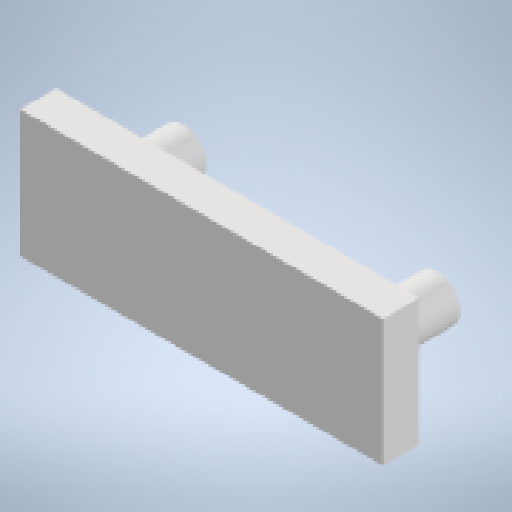
# Autodesk Inventor part: test_izbrisi
Saved by Autodesk Inventor 2023 (Build 270158000, 158)
## iProperties
Created: 2022-09-28
Part Number: test_izbrisi
Material: Generic
Document SubType Name: Modeling
Designer: simon
Density: 1 g/cm^3
Appearance: Default
Author: simon
Autodesk Inventor part; units mm, degrees
ref_plane "YZ Plane" through (0, 0, 0) normal (1, 0, 0) x (0, 1, 0)
ref_plane "XZ Plane" through (0, 0, 0) normal (0, 1, 0) x (-1, 0, 0)
ref_plane "XY Plane" through (0, 0, 0) normal (0, 0, 1) x (1, 0, 0)
sketch "Sketch2" plane through (0, 0, 0) normal (0, 0, 1) x (1, 0, 0)
  circle A0 centre (14, 0) radius 1.25 projected
  circle A1 centre (0, 0) radius 1.25 projected
  line L0 (-3, -3.5) -> (17, -3.5) projected
  line L1 (17, -3.5) -> (17, 3.5) projected
  line L2 (17, 3.5) -> (-3, 3.5) projected
  line L3 (-3, 3.5) -> (-3, -3.5) projected
extrude "Extrusion1" add sketch "Sketch2" along normal blind 2 contours A0 | A1 | L3 L2 L1 L0
extrude "Extrusion2" add sketch "Sketch2" against normal blind 4 contours A0 | A1
body "Solid1"
